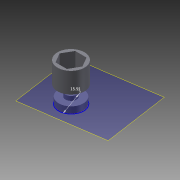
# Autodesk Inventor part: SmallGearOutput
Saved by Autodesk Inventor 2012 (Build 160160000, 160)
## iProperties
Created: 2011-10-22
Part Number: SmallGearOutput
Material: Steel
Document SubType Name: Modeling
Designer: KuttaA
Categories: <?xml version="1.0" encoding="UTF-16"?> <MemberInstance><Categories><FamilyTemplate><FamilyTemplateParameter ValueType="xs:double" Id="1" ObjectReferenceKey="da_z" ObjectType="kUserParameterObject"/><FamilyTemplateParameter ValueType="xs:double" Id="2" ObjectReferenceKey="da_b" ObjectType="kUserParameterObject"/><FamilyTemplateParameter ValueType="xs:double" Id="3" ObjectReferenceKey="da_beta" ObjectType="kUserParameterObject"/><FamilyTemplateParameter ValueType="xs:double" Id="4" ObjectReferenceKey="da_da" ObjectType="kUserParameterObject"/><FamilyTemplateParameter ValueType="xs:double" Id="5" ObjectReferenceKey="da_aw" ObjectType="kUserParameterObject"/><FamilyTemplateParameter ValueType="xs:string" Id="6" ObjectReferenceKey="EAIAABAAAACIAQAAAAAAAIAAAAAAAAAA" ObjectType="83910656" SubObjectId="SurfaceGeometry"/></FamilyTemplate><ParamToTemplateMap><ParamToTemplate CategoryParameter="//CategoryParameter[@InternalName='046C89C9-8512-4d59-83FE-43B91F4F132A']" TemplateParameter="1"/><ParamToTemplate CategoryParameter="//CategoryParameter[@InternalName='2552DF32-E462-4b46-AEBF-C6C7768E72AC']" TemplateParameter="2"/><ParamToTemplate CategoryParameter="//CategoryParameter[@InternalName='C9EE641D-15FC-4fae-A226-E94C4372FDD7']" TemplateParameter="3"/><ParamToTemplate><ParamToTemplate CategoryParameter="//CategoryParameter[@InternalName='00B6519A-459B-49c7-AD84-2E56D39A5744']" ConstantValue="0.000000"/></ParamToTemplate><ParamToTemplate><ParamToTemplate CategoryParameter="//CategoryParameter[@InternalName='04B31F0E-C7A6-4894-AA32-9629BEFACF47']" ConstantValue="1.000000"/></ParamToTemplate><ParamToTemplate><ParamToTemplate CategoryParameter="//CategoryParameter[@InternalName='43CBEC2E-7847-49e7-A936-2F7889FCB2D9']" ConstantValue="0.250000"/></ParamToTemplate><ParamToTemplate><ParamToTemplate CategoryParameter="//CategoryParameter[@InternalName='B1EFC894-105D-4ebd-86BF-FA20ED196853']" ConstantValue="0.302500"/></ParamToTemplate><ParamToTemplate><ParamToTemplate CategoryParameter="//CategoryParameter[@InternalName='51175063-3D10-4879-93E8-6246FE8B403D']" ConstantValue="2060000000.000000"/></ParamToTemplate><ParamToTemplate><ParamToTemplate CategoryParameter="//CategoryParameter[@InternalName='A3A52E27-4454-46a9-B0BD-C932399B70AF']" ConstantValue="0.300000"/></ParamToTemplate><ParamToTemplate><ParamToTemplate CategoryParameter="//CategoryParameter[@InternalName='91B76062-C214-41d9-B1B9-14D2AB99603D']" ConstantValue="0.031750"/></ParamToTemplate><ParamToTemplate><ParamToTemplate CategoryParameter="//CategoryParameter[@InternalName='374E806E-8B8A-4dda-A9AA-1039D6500AD2']" ConstantValue="31.496063"/></ParamToTemplate><ParamToTemplate><ParamToTemplate CategoryParameter="//CategoryParameter[@InternalName='2D373A89-B862-43d6-8D0B-0CBF12AB9F6C']" ConstantValue="0.349066"/></ParamToTemplate><ParamToTemplate CategoryParameter="//CategoryParameter[@InternalName='37777632-D6A2-4fac-9D53-DB8ACD95C989']" TemplateParameter="4"/><ParamToTemplate CategoryParameter="//CategoryParameter[@InternalName='FD1017F1-B727-4f7e-9707-0F86F1FF9423']" TemplateParameter="5"/><ParamToTemplate><ParamToTemplate CategoryParameter="//CategoryParameter[@InternalName='9E1B4470-B2D3-4ff1-B813-535BB4CDF51A']" ConstantValue="3520000.000000"/></ParamToTemplate><ParamToTemplate><ParamToTemplate CategoryParameter="//CategoryParameter[@InternalName='F8452263-BFF6-458c-9FB1-07C4B99E95CD']" ConstantValue="11400000.000000"/></ParamToTemplate><ParamToTemplate><ParamToTemplate CategoryParameter="//CategoryParameter[@InternalName='3E3BB259-FD49-497f-8171-6EBC954A3479']" ConstantValue="2.000000"/></ParamToTemplate><ParamToTemplate CategoryParameter="//CategoryParameter[@InternalName='27C3BAF2-7550-4e4b-AE2C-0DB134B7D9B7']" TemplateParameter="6"/></ParamToTemplateMap><Category DisplayName="Gear" InternalName="DC85795E-93AB-48d5-8EEE-5A27447B64BD" Mnemonic="Gear"><CategoryParameter DisplayName="z" InternalName="046C89C9-8512-4d59-83FE-43B91F4F132A" Mnemonic="z"/><CategoryParameter DisplayName="b" InternalName="2552DF32-E462-4b46-AEBF-C6C7768E72AC" Mnemonic="b"/><CategoryParameter DisplayName="||b|" InternalName="C9EE641D-15FC-4fae-A226-E94C4372FDD7" Mnemonic="beta"/><CategoryParameter DisplayName="x" InternalName="00B6519A-459B-49c7-AD84-2E56D39A5744" Mnemonic="x"/><CategoryParameter DisplayName="a*" InternalName="04B31F0E-C7A6-4894-AA32-9629BEFACF47" Mnemonic="a"/><CategoryParameter DisplayName="c*" InternalName="43CBEC2E-7847-49e7-A936-2F7889FCB2D9" Mnemonic="c"/><CategoryParameter DisplayName="r|.f|*" InternalName="B1EFC894-105D-4ebd-86BF-FA20ED196853" Mnemonic="rf"/><CategoryParameter DisplayName="E" InternalName="51175063-3D10-4879-93E8-6246FE8B403D" Mnemonic="E"/><CategoryParameter DisplayName="||m|" InternalName="A3A52E27-4454-46a9-B0BD-C932399B70AF" Mnemonic="mi"/><Category DisplayName="SpurGear" InternalName="26C5A22E-A91E-4dfd-A3B3-23CCAFAE1764" Mnemonic="SpurGear"><CategoryParameter DisplayName="m" InternalName="91B76062-C214-41d9-B1B9-14D2AB99603D" Mnemonic="m"/><CategoryParameter DisplayName="P" InternalName="374E806E-8B8A-4dda-A9AA-1039D6500AD2" Mnemonic="PP"/><CategoryParameter DisplayName="||a|" InternalName="2D373A89-B862-43d6-8D0B-0CBF12AB9F6C" Mnemonic="alpha"/><CategoryParameter DisplayName="d|.a|" InternalName="37777632-D6A2-4fac-9D53-DB8ACD95C989" Mnemonic="da"/><CategoryParameter DisplayName="a|.w|" InternalName="FD1017F1-B727-4f7e-9707-0F86F1FF9423" Mnemonic="aw"/><CategoryParameter DisplayName="||s||.Flim|" InternalName="9E1B4470-B2D3-4ff1-B813-535BB4CDF51A" Mnemonic="sFlim"/><CategoryParameter DisplayName="||s||.Hlim|" InternalName="F8452263-BFF6-458c-9FB1-07C4B99E95CD" Mnemonic="sHlim"/><CategoryParameter DisplayName="type" InternalName="3E3BB259-FD49-497f-8171-6EBC954A3479" Mnemonic="type"/><CategoryParameter DisplayName="PitchDiameter" InternalName="27C3BAF2-7550-4e4b-AE2C-0DB134B7D9B7" Mnemonic="IDS_PITCHDIAM"/></Category></Category></Categories></MemberInstance>
Density: 7.85 g/cm^3
Mass: 19.4399 g
Surface Area: 23.9063 cm^2
Volume: 2.47642 cm^3
CustomPartVersion: 1
Author: KuttaA
Autodesk Inventor part; units mm, degrees
ref_plane "YZ Plane" through (0, 0, 0) normal (1, 0, 0) x (0, 1, 0)
ref_plane "XZ Plane" through (0, 0, 0) normal (0, 1, 0) x (-1, 0, 0)
ref_plane "XY Plane" through (0, 0, 0) normal (0, 0, 1) x (1, 0, 0)
sketch "Sketch1" plane through (0, 0, 0) normal (0, 0, 1) x (1, 0, 0)
  circle A0 centre (0, 0) radius 7.7508
  dimension "d0" = 15.5016
  constraints: 1 centre point
  measures "d0" diameter of A0
extrude "Extrusion1" add sketch "Sketch1" along normal blind 4
ref_plane "Work Plane2" through (0, 0, 2) normal (0, 0, 1) x (1, 0, 0)
sketch "Sketch2" plane through (0, 0, 0) normal (0, 0, -1) x (-1, 0, 0)
  circle A0 centre (0, 0) radius 7.7508 projected
  circle A1 centre (0, 0) radius 7.4314
  dimension "d3" = 14.8628
  constraints: 1 centre point, 1 coincident
  measures "d3" diameter of A1
surface extrude "Pitch Diameter" sketch "Sketch2" against normal through all shown no curves A1
ref_plane "Work Plane8" through (0, 0, 0) normal (0.9974521, 0.0713392, 0) x (0, 0, 1)
ref_plane "Work Plane9" through (0, 0, 0) normal (1, 0, 0) x (0, 1, 0)
feature "Spur Gear" [suppressed]
sketch "Sketch4" plane through (0, 0, 4) normal (0, 0, 1) x (1, 0, 0)
  circle A0 centre (0, 0) radius 2.5
  dimension "d52" = 5
  constraints: 1 centre point, 1 coincident
  measures "d52" diameter of A0
extrude "Extrusion3" add sketch "Sketch4" along normal blind 10
sketch "Sketch5" plane through (0, 0, 14) normal (0, 0, 1) x (1, 0, 0)
  circle A0 centre (0, 0) radius 2.5 construction
  circle A1 centre (0, 0) radius 8.5
  line L0 (-3.6084, 6.25) -> (3.6084, 6.25)
  line L1 (3.6084, 6.25) -> (7.2169, 0)
  line L2 (7.2169, 0) -> (3.6106, -6.2513)
  line L3 (3.6106, -6.2513) -> (-3.6062, -6.2513)
  line L4 (-3.6062, -6.2513) -> (-7.2147, -0.0013)
  line L5 (-7.2147, -0.0013) -> (-3.6084, 6.25)
  line L6 (0, 0) -> (-3.6062, -6.2513) construction
  line L7 (0, 0) -> (-3.6084, 6.25) construction
  line L8 (0, 0) -> (3.6084, 6.25) construction
  line L9 (0, 0) -> (7.2169, 0) construction
  dimension "d56" = 17
  dimension "d57" = 12.5
  constraints: 20 end point, 6 equal length, 4 parallel, 1 centre point, 1 coincident, 1 horizontal
  measures "d56" diameter of A1
  measures "d57" distance between parallel lines of L2 L5
extrude "Extrusion4" add sketch "Sketch5" along normal blind 10
sketch "Sketch6" plane through (0, 0, 14) normal (0, 0, -1) x (-1, 0, 0)
  circle A0 centre (0, 0) radius 8.5 projected
extrude "Extrusion5" add sketch "Sketch6" along normal blind 3
ref_plane "Work Plane11" through (9.0258, 1.3096, 7) normal (0, 0, -1) x (0.989584, 0.1439567, 0)
sketch "Sketch7" plane through (9.0258, 1.3096, 7) normal (0, 0, -1) x (0.989584, 0.1439567, 0)
  circle A0 centre (-9.1203, -0.0034) radius 2.5 projected
  circle A1 centre (-9.1203, -0.0034) radius 2.5 projected
  circle A2 centre (-9.1203, -0.0034) radius 3.5
  point P0 (-9.1203, -0.0034)
  dimension "d62" = 1
  constraints: 1 centre point, 1 coincident
  measures "d62" radial gap between concentric circles of A2 A0
extrude "Extrusion6" add sketch "Sketch7" along normal blind 3
sketch "Sketch8" plane through (0, 0, 7) normal (0, 0, 1) x (1, 0, 0)
  circle A0 centre (0, 0) radius 3.5 projected
  circle A1 centre (0, 0) radius 2.5 projected
  point P0 (0, 0)
extrude "Extrusion7" cut sketch "Sketch8" against normal blind 0.3
sketch "Sketch9" plane through (0, 0, 0) normal (0, 0, -1) x (-1, 0, 0)
  arc A0 (1.3727, 6.9012) -> (-7.7508, 0) centre (-7.7508, 0) ccw construction
  arc A1 (-7.7508, 0) -> (-7.7508, 0) centre (0, 0) ccw construction
  arc A2 (-7.7508, 0) -> (0.6272, 7.0084) centre (0.6272, 7.0084) ccw construction
  arc A3 (0.6272, 7.0084) -> (0.3766, 7.0263) centre (0.3766, 7.0263) ccw construction
  arc A4 (0.3766, 7.0263) -> (-7.7508, 0) centre (-7.7508, 0) ccw construction
  arc A5 (-7.7508, 0) -> (-7.7508, 0) centre (0, 0) ccw construction
  arc A6 (-7.7508, 0) -> (-0.3766, 7.0263) centre (-0.3766, 7.0263) ccw construction
  arc A7 (-0.3766, 7.0263) -> (-0.6272, 7.0084) centre (-0.6272, 7.0084) ccw construction
  arc A8 (-0.6272, 7.0084) -> (-7.7508, 0) centre (-7.7508, 0) ccw construction
  arc A9 (-7.7508, 0) -> (-7.7508, 0) centre (0, 0) ccw construction
  arc A10 (-7.7508, 0) -> (-1.3727, 6.9012) centre (-1.3727, 6.9012) ccw construction
  arc A11 (-1.3727, 6.9012) -> (-1.6182, 6.8478) centre (-1.6182, 6.8478) ccw construction
  arc A12 (-1.6182, 6.8478) -> (-7.7508, 0) centre (-7.7508, 0) ccw construction
  arc A13 (-7.7508, 0) -> (-7.7508, 0) centre (0, 0) ccw construction
  arc A14 (-7.7508, 0) -> (-2.3409, 6.6356) centre (-2.3409, 6.6356) ccw construction
  arc A15 (-2.3409, 6.6356) -> (-2.5763, 6.5478) centre (-2.5763, 6.5478) ccw construction
  arc A16 (-2.5763, 6.5478) -> (-7.7508, 0) centre (-7.7508, 0) ccw construction
  arc A17 (-7.7508, 0) -> (-7.7508, 0) centre (0, 0) ccw construction
  arc A18 (-7.7508, 0) -> (-3.2614, 6.2349) centre (-3.2614, 6.2349) ccw construction
  arc A19 (-3.2614, 6.2349) -> (-3.4819, 6.1145) centre (-3.4819, 6.1145) ccw construction
  arc A20 (-3.4819, 6.1145) -> (-7.7508, 0) centre (-7.7508, 0) ccw construction
  arc A21 (-7.7508, 0) -> (-7.7508, 0) centre (0, 0) ccw construction
  arc A22 (-7.7508, 0) -> (-4.1155, 5.7073) centre (-4.1155, 5.7073) ccw construction
  arc A23 (-4.1155, 5.7073) -> (-4.3166, 5.5568) centre (-4.3166, 5.5568) ccw construction
  arc A24 (-4.3166, 5.5568) -> (-7.7508, 0) centre (-7.7508, 0) ccw construction
  arc A25 (-7.7508, 0) -> (-7.7508, 0) centre (0, 0) ccw construction
  arc A26 (-7.7508, 0) -> (-4.8859, 5.0635) centre (-4.8859, 5.0635) ccw construction
  arc A27 (-4.8859, 5.0635) -> (-5.0635, 4.8859) centre (-5.0635, 4.8859) ccw construction
  arc A28 (-5.0635, 4.8859) -> (-7.7508, 0) centre (-7.7508, 0) ccw construction
  arc A29 (-7.7508, 0) -> (-7.7508, 0) centre (0, 0) ccw construction
  arc A30 (-7.7508, 0) -> (-5.5568, 4.3166) centre (-5.5568, 4.3166) ccw construction
  arc A31 (-5.5568, 4.3166) -> (-5.7073, 4.1155) centre (-5.7073, 4.1155) ccw construction
  arc A32 (-5.7073, 4.1155) -> (-7.7508, 0) centre (-7.7508, 0) ccw construction
  arc A33 (-7.7508, 0) -> (-7.7508, 0) centre (0, 0) ccw construction
  arc A34 (-7.7508, 0) -> (-6.1145, 3.4819) centre (-6.1145, 3.4819) ccw construction
  arc A35 (-6.1145, 3.4819) -> (-6.2349, 3.2614) centre (-6.2349, 3.2614) ccw construction
  arc A36 (-6.2349, 3.2614) -> (-7.7508, 0) centre (-7.7508, 0) ccw construction
  arc A37 (-7.7508, 0) -> (-7.7508, 0) centre (0, 0) ccw construction
  arc A38 (-7.7508, 0) -> (-6.5478, 2.5763) centre (-6.5478, 2.5763) ccw construction
  arc A39 (-6.5478, 2.5763) -> (-6.6356, 2.3409) centre (-6.6356, 2.3409) ccw construction
  arc A40 (-6.6356, 2.3409) -> (-7.7508, 0) centre (-7.7508, 0) ccw construction
  arc A41 (-7.7508, 0) -> (-7.7508, 0) centre (0, 0) ccw construction
  arc A42 (-7.7508, 0) -> (-6.8478, 1.6182) centre (-6.8478, 1.6182) ccw construction
  arc A43 (-6.8478, 1.6182) -> (-6.9012, 1.3727) centre (-6.9012, 1.3727) ccw construction
  arc A44 (-6.9012, 1.3727) -> (-7.7508, 0) centre (-7.7508, 0) ccw construction
  arc A45 (-7.7508, 0) -> (-7.7508, 0) centre (0, 0) ccw construction
  arc A46 (-7.7508, 0) -> (-7.0084, 0.6272) centre (-7.0084, 0.6272) ccw construction
  arc A47 (-7.0084, 0.6272) -> (-7.0263, 0.3766) centre (-7.0263, 0.3766) ccw construction
  arc A48 (-7.0263, 0.3766) -> (-7.7508, 0) centre (-7.7508, 0) ccw construction
  arc A49 (-7.7508, 0) -> (-7.7508, 0) centre (0, 0) ccw construction
  arc A50 (-7.7508, 0) -> (-7.0263, -0.3766) centre (-7.0263, -0.3766) ccw construction
  arc A51 (-7.0263, -0.3766) -> (-7.0084, -0.6272) centre (-7.0084, -0.6272) ccw construction
  arc A52 (-7.0084, -0.6272) -> (-7.7508, 0) centre (-7.7508, 0) ccw construction
  arc A53 (-7.7508, 0) -> (-7.7508, 0) centre (0, 0) ccw construction
  arc A54 (-7.7508, 0) -> (-6.9012, -1.3727) centre (-6.9012, -1.3727) ccw construction
  arc A55 (-6.9012, -1.3727) -> (-6.8478, -1.6182) centre (-6.8478, -1.6182) ccw construction
  arc A56 (-6.8478, -1.6182) -> (-7.7508, 0) centre (-7.7508, 0) ccw construction
  arc A57 (-7.7508, 0) -> (-7.7508, 0) centre (0, 0) ccw construction
  arc A58 (-7.7508, 0) -> (-6.6356, -2.3409) centre (-6.6356, -2.3409) ccw construction
  arc A59 (-6.6356, -2.3409) -> (-6.5478, -2.5763) centre (-6.5478, -2.5763) ccw construction
  arc A60 (-6.5478, -2.5763) -> (-7.7508, 0) centre (-7.7508, 0) ccw construction
  arc A61 (-7.7508, 0) -> (-7.7508, 0) centre (0, 0) ccw construction
  arc A62 (-7.7508, 0) -> (-6.2349, -3.2614) centre (-6.2349, -3.2614) ccw construction
  arc A63 (-6.2349, -3.2614) -> (-6.1145, -3.4819) centre (-6.1145, -3.4819) ccw construction
  arc A64 (-6.1145, -3.4819) -> (-7.7508, 0) centre (-7.7508, 0) ccw construction
  arc A65 (-7.7508, 0) -> (-7.7508, 0) centre (0, 0) ccw construction
  arc A66 (-7.7508, 0) -> (-5.7073, -4.1155) centre (-5.7073, -4.1155) ccw construction
  arc A67 (-5.7073, -4.1155) -> (-5.5568, -4.3166) centre (-5.5568, -4.3166) ccw construction
  arc A68 (-5.5568, -4.3166) -> (-7.7508, 0) centre (-7.7508, 0) ccw construction
  arc A69 (-7.7508, 0) -> (-7.7508, 0) centre (0, 0) ccw construction
  arc A70 (-7.7508, 0) -> (-5.0635, -4.8859) centre (-5.0635, -4.8859) ccw construction
  arc A71 (-5.0635, -4.8859) -> (-4.8859, -5.0635) centre (-4.8859, -5.0635) ccw construction
  arc A72 (-4.8859, -5.0635) -> (-7.7508, 0) centre (-7.7508, 0) ccw construction
  arc A73 (-7.7508, 0) -> (-7.7508, 0) centre (0, 0) ccw construction
  arc A74 (-7.7508, 0) -> (-4.3166, -5.5568) centre (-4.3166, -5.5568) ccw construction
  arc A75 (-4.3166, -5.5568) -> (-4.1155, -5.7073) centre (-4.1155, -5.7073) ccw construction
  arc A76 (-4.1155, -5.7073) -> (-7.7508, 0) centre (-7.7508, 0) ccw construction
  arc A77 (-7.7508, 0) -> (-7.7508, 0) centre (0, 0) ccw construction
  arc A78 (-7.7508, 0) -> (-3.4819, -6.1145) centre (-3.4819, -6.1145) ccw construction
  arc A79 (-3.4819, -6.1145) -> (-3.2614, -6.2349) centre (-3.2614, -6.2349) ccw construction
  arc A80 (-3.2614, -6.2349) -> (-7.7508, 0) centre (-7.7508, 0) ccw construction
  arc A81 (-7.7508, 0) -> (-7.7508, 0) centre (0, 0) ccw construction
  arc A82 (-7.7508, 0) -> (-2.5763, -6.5478) centre (-2.5763, -6.5478) ccw construction
  arc A83 (-2.5763, -6.5478) -> (-2.3409, -6.6356) centre (-2.3409, -6.6356) ccw construction
  arc A84 (-2.3409, -6.6356) -> (-7.7508, 0) centre (-7.7508, 0) ccw construction
  arc A85 (-7.7508, 0) -> (-7.7508, 0) centre (0, 0) ccw construction
  arc A86 (-7.7508, 0) -> (-1.6182, -6.8478) centre (-1.6182, -6.8478) ccw construction
  arc A87 (-1.6182, -6.8478) -> (-1.3727, -6.9012) centre (-1.3727, -6.9012) ccw construction
  arc A88 (-1.3727, -6.9012) -> (-7.7508, 0) centre (-7.7508, 0) ccw construction
  arc A89 (-7.7508, 0) -> (-7.7508, 0) centre (0, 0) ccw construction
  arc A90 (-7.7508, 0) -> (-0.6272, -7.0084) centre (-0.6272, -7.0084) ccw construction
  arc A91 (-0.6272, -7.0084) -> (-0.3766, -7.0263) centre (-0.3766, -7.0263) ccw construction
  arc A92 (-0.3766, -7.0263) -> (-7.7508, 0) centre (-7.7508, 0) ccw construction
  arc A93 (-7.7508, 0) -> (-7.7508, 0) centre (0, 0) ccw construction
  arc A94 (-7.7508, 0) -> (0.3766, -7.0263) centre (0.3766, -7.0263) ccw construction
  arc A95 (0.3766, -7.0263) -> (0.6272, -7.0084) centre (0.6272, -7.0084) ccw construction
  arc A96 (0.6272, -7.0084) -> (-7.7508, 0) centre (-7.7508, 0) ccw construction
  arc A97 (-7.7508, 0) -> (-7.7508, 0) centre (0, 0) ccw construction
  arc A98 (-7.7508, 0) -> (1.3727, -6.9012) centre (1.3727, -6.9012) ccw construction
  arc A99 (1.3727, -6.9012) -> (1.6182, -6.8478) centre (1.6182, -6.8478) ccw construction
  arc A100 (1.6182, -6.8478) -> (-7.7508, 0) centre (-7.7508, 0) ccw construction
  arc A101 (-7.7508, 0) -> (-7.7508, 0) centre (0, 0) ccw construction
  arc A102 (-7.7508, 0) -> (2.3409, -6.6356) centre (2.3409, -6.6356) ccw construction
  arc A103 (2.3409, -6.6356) -> (2.5763, -6.5478) centre (2.5763, -6.5478) ccw construction
  arc A104 (2.5763, -6.5478) -> (-7.7508, 0) centre (-7.7508, 0) ccw construction
  arc A105 (-7.7508, 0) -> (-7.7508, 0) centre (0, 0) ccw construction
  arc A106 (-7.7508, 0) -> (3.2614, -6.2349) centre (3.2614, -6.2349) ccw construction
  arc A107 (3.2614, -6.2349) -> (3.4819, -6.1145) centre (3.4819, -6.1145) ccw construction
  arc A108 (3.4819, -6.1145) -> (-7.7508, 0) centre (-7.7508, 0) ccw construction
  arc A109 (-7.7508, 0) -> (-7.7508, 0) centre (0, 0) ccw construction
  arc A110 (-7.7508, 0) -> (4.1155, -5.7073) centre (4.1155, -5.7073) ccw construction
  arc A111 (4.1155, -5.7073) -> (4.3166, -5.5568) centre (4.3166, -5.5568) ccw construction
  arc A112 (4.3166, -5.5568) -> (-7.7508, 0) centre (-7.7508, 0) ccw construction
  arc A113 (-7.7508, 0) -> (-7.7508, 0) centre (0, 0) ccw construction
  arc A114 (-7.7508, 0) -> (4.8859, -5.0635) centre (4.8859, -5.0635) ccw construction
  arc A115 (4.8859, -5.0635) -> (5.0635, -4.8859) centre (5.0635, -4.8859) ccw construction
  arc A116 (5.0635, -4.8859) -> (-7.7508, 0) centre (-7.7508, 0) ccw construction
  arc A117 (-7.7508, 0) -> (-7.7508, 0) centre (0, 0) ccw construction
  arc A118 (-7.7508, 0) -> (5.5568, -4.3166) centre (5.5568, -4.3166) ccw construction
  arc A119 (5.5568, -4.3166) -> (5.7073, -4.1155) centre (5.7073, -4.1155) ccw construction
  arc A120 (5.7073, -4.1155) -> (-7.7508, 0) centre (-7.7508, 0) ccw construction
  arc A121 (-7.7508, 0) -> (-7.7508, 0) centre (0, 0) ccw construction
  arc A122 (-7.7508, 0) -> (6.1145, -3.4819) centre (6.1145, -3.4819) ccw construction
  arc A123 (6.1145, -3.4819) -> (6.2349, -3.2614) centre (6.2349, -3.2614) ccw construction
  arc A124 (6.2349, -3.2614) -> (-7.7508, 0) centre (-7.7508, 0) ccw construction
  arc A125 (-7.7508, 0) -> (-7.7508, 0) centre (0, 0) ccw construction
  arc A126 (-7.7508, 0) -> (6.5478, -2.5763) centre (6.5478, -2.5763) ccw construction
  arc A127 (6.5478, -2.5763) -> (6.6356, -2.3409) centre (6.6356, -2.3409) ccw construction
  arc A128 (6.6356, -2.3409) -> (-7.7508, 0) centre (-7.7508, 0) ccw construction
  arc A129 (-7.7508, 0) -> (-7.7508, 0) centre (0, 0) ccw construction
  arc A130 (-7.7508, 0) -> (6.8478, -1.6182) centre (6.8478, -1.6182) ccw construction
  arc A131 (6.8478, -1.6182) -> (6.9012, -1.3727) centre (6.9012, -1.3727) ccw construction
  arc A132 (6.9012, -1.3727) -> (-7.7508, 0) centre (-7.7508, 0) ccw construction
  arc A133 (-7.7508, 0) -> (-7.7508, 0) centre (0, 0) ccw construction
  arc A134 (-7.7508, 0) -> (7.0084, -0.6272) centre (7.0084, -0.6272) ccw construction
  arc A135 (7.0084, -0.6272) -> (7.0263, -0.3766) centre (7.0263, -0.3766) ccw construction
  arc A136 (7.0263, -0.3766) -> (-7.7508, 0) centre (-7.7508, 0) ccw construction
  arc A137 (-7.7508, 0) -> (-7.7508, 0) centre (0, 0) ccw construction
  arc A138 (-7.7508, 0) -> (7.0263, 0.3766) centre (7.0263, 0.3766) ccw construction
  arc A139 (7.0263, 0.3766) -> (7.0084, 0.6272) centre (7.0084, 0.6272) ccw construction
  arc A140 (7.0084, 0.6272) -> (-7.7508, 0) centre (-7.7508, 0) ccw construction
  arc A141 (-7.7508, 0) -> (-7.7508, 0) centre (0, 0) ccw construction
  arc A142 (-7.7508, 0) -> (6.9012, 1.3727) centre (6.9012, 1.3727) ccw construction
  arc A143 (6.9012, 1.3727) -> (6.8478, 1.6182) centre (6.8478, 1.6182) ccw construction
  arc A144 (6.8478, 1.6182) -> (-7.7508, 0) centre (-7.7508, 0) ccw construction
  arc A145 (-7.7508, 0) -> (-7.7508, 0) centre (0, 0) ccw construction
  arc A146 (-7.7508, 0) -> (6.6356, 2.3409) centre (6.6356, 2.3409) ccw construction
  arc A147 (6.6356, 2.3409) -> (6.5478, 2.5763) centre (6.5478, 2.5763) ccw construction
  arc A148 (6.5478, 2.5763) -> (-7.7508, 0) centre (-7.7508, 0) ccw construction
  arc A149 (-7.7508, 0) -> (-7.7508, 0) centre (0, 0) ccw construction
  arc A150 (-7.7508, 0) -> (6.2349, 3.2614) centre (6.2349, 3.2614) ccw construction
  arc A151 (6.2349, 3.2614) -> (6.1145, 3.4819) centre (6.1145, 3.4819) ccw construction
  arc A152 (6.1145, 3.4819) -> (-7.7508, 0) centre (-7.7508, 0) ccw construction
  arc A153 (-7.7508, 0) -> (-7.7508, 0) centre (0, 0) ccw construction
  arc A154 (-7.7508, 0) -> (5.7073, 4.1155) centre (5.7073, 4.1155) ccw construction
  arc A155 (5.7073, 4.1155) -> (5.5568, 4.3166) centre (5.5568, 4.3166) ccw construction
  arc A156 (5.5568, 4.3166) -> (-7.7508, 0) centre (-7.7508, 0) ccw construction
  arc A157 (-7.7508, 0) -> (-7.7508, 0) centre (0, 0) ccw construction
  arc A158 (-7.7508, 0) -> (5.0635, 4.8859) centre (5.0635, 4.8859) ccw construction
  arc A159 (5.0635, 4.8859) -> (4.8859, 5.0635) centre (4.8859, 5.0635) ccw construction
  arc A160 (4.8859, 5.0635) -> (-7.7508, 0) centre (-7.7508, 0) ccw construction
  arc A161 (-7.7508, 0) -> (-7.7508, 0) centre (0, 0) ccw construction
  arc A162 (-7.7508, 0) -> (4.3166, 5.5568) centre (4.3166, 5.5568) ccw construction
  arc A163 (4.3166, 5.5568) -> (4.1155, 5.7073) centre (4.1155, 5.7073) ccw construction
  arc A164 (4.1155, 5.7073) -> (-7.7508, 0) centre (-7.7508, 0) ccw construction
  arc A165 (-7.7508, 0) -> (-7.7508, 0) centre (0, 0) ccw construction
  arc A166 (-7.7508, 0) -> (3.4819, 6.1145) centre (3.4819, 6.1145) ccw construction
  arc A167 (3.4819, 6.1145) -> (3.2614, 6.2349) centre (3.2614, 6.2349) ccw construction
  arc A168 (3.2614, 6.2349) -> (-7.7508, 0) centre (-7.7508, 0) ccw construction
  arc A169 (-7.7508, 0) -> (-7.7508, 0) centre (0, 0) ccw construction
  arc A170 (-7.7508, 0) -> (2.5763, 6.5478) centre (2.5763, 6.5478) ccw construction
  arc A171 (2.5763, 6.5478) -> (2.3409, 6.6356) centre (2.3409, 6.6356) ccw construction
  arc A172 (2.3409, 6.6356) -> (-7.7508, 0) centre (-7.7508, 0) ccw construction
  arc A173 (-7.7508, 0) -> (-7.7508, 0) centre (0, 0) ccw construction
  arc A174 (-7.7508, 0) -> (1.6182, 6.8478) centre (1.6182, 6.8478) ccw construction
  arc A175 (1.6182, 6.8478) -> (1.3727, 6.9012) centre (1.3727, 6.9012) ccw construction
  circle A176 centre (0, 0) radius 7.955
  dimension "d67" = 15.9099
  constraints: 1 centre point, 1 coincident, 132 other
  measures "d67" diameter of A176
equation "\"d0\" = da_da"
equation "\"d1\" = da_b"
equation "\"d3\" = da_dw"
equation "\"d16\" = da_aw"
equation "\"d43\" = da_aw"
equation "\"d46\" = da_aw"
equation "\"da_da\" = 15.501556"
equation "\"da_b\" = 4"
equation "\"da_dw\" = 14.86278"
equation "\"da_aw\" = 18.071789"
body "Solid1"
body "Srf1"
